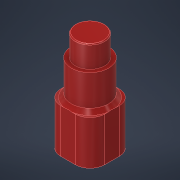
# Autodesk Inventor part: CH_01_0020_servo_shaft_1
Saved by Autodesk Inventor 2022 (Build 260153000, 153)
## iProperties
Created: 2022-03-04
Part Number: CH_01_0020_servo_shaft_1
Material: Ogólny
Document SubType Name: Modeling
Designer: zsamot8
Density: 1 g/cm^3
Appearance: Czerwona
Author: zsamot8
Autodesk Inventor part; units mm, degrees
ref_plane "YZ Plane" through (0, 0, 0) normal (1, 0, 0) x (0, 1, 0)
ref_plane "XZ Plane" through (0, 0, 0) normal (0, 1, 0) x (-1, 0, 0)
ref_plane "XY Plane" through (0, 0, 0) normal (0, 0, 1) x (1, 0, 0)
sketch "Szkic1" plane through (0, 0, 0) normal (0, 1, 0) x (-1, 0, 0)
  line L0 (-2.75, 2.75) -> (2.75, 2.75)
  line L1 (2.75, 2.75) -> (2.75, -2.75)
  line L2 (2.75, -2.75) -> (-2.75, -2.75)
  line L3 (-2.75, -2.75) -> (-2.75, 2.75)
  line L4 (-2.75, 2.75) -> (2.75, -2.75) construction
  line L5 (2.75, 2.75) -> (-2.75, -2.75) construction
  line L6 (-2, 6) -> (2, 6)
  line L7 (6, 2) -> (6, -2)
  line L8 (2, -6) -> (-2, -6)
  line L9 (-6, -2) -> (-6, 2)
  line L10 (-6, 6) -> (6, -6) construction
  line L11 (6, 6) -> (-6, -6) construction
  arc A0 (6, 2) -> (2, 6) centre (2, 2) ccw
  arc A1 (2, -6) -> (6, -2) centre (2, -2) ccw
  arc A2 (-6, -2) -> (-2, -6) centre (-2, -2) ccw
  arc A3 (-2, 6) -> (-6, 2) centre (-2, 2) ccw
  point P0 (0, 0)
  dimension "d0" = 5.5
  dimension "d1" = 12
  dimension "d2" = 4
  constraints: 24 end point, 9 point on line, 8 point on circle, 8 tangent, 4 centre point, 4 midpoint, 4 parallel, 3 equal radius, 3 perpendicular, 2 horizontal
  measures "d0" distance between parallel lines of L2 L0
  measures "d1" distance of L11.start L10.end
  measures "d2" radius of A0
extrude "Wyciągnięcie proste1" add sketch "Szkic1" along normal blind 10
sketch "Szkic2" plane through (0, 10, 0) normal (0, 1, 0) x (1, 0, 0)
  arc A0 (-6, -2) -> (-2, -6) centre (-2, -2) ccw projected
  line L0 (-6, 2) -> (-6, -2) projected
  arc A1 (-2, 6) -> (-6, 2) centre (-2, 2) ccw projected
  line L1 (2, 6) -> (-2, 6) projected
  arc A2 (6, 2) -> (2, 6) centre (2, 2) ccw projected
  line L2 (6, -2) -> (6, 2) projected
  arc A3 (2, -6) -> (6, -2) centre (2, -2) ccw projected
  line L3 (-2, -6) -> (2, -6) projected
extrude "Wyciągnięcie proste2" add sketch "Szkic2" along normal blind 2
sketch "Szkic3" plane through (0, 12, 0) normal (0, 1, 0) x (1, 0, 0)
  circle A0 centre (0, 0) radius 4
  dimension "d7" = 8
  constraints: 1 centre point, 1 coincident
  measures "d7" diameter of A0
extrude "Wyciągnięcie proste3" add sketch "Szkic3" along normal blind 15.45
sketch "Szkic5" plane through (0, 12, 0) normal (0, 1, 0) x (1, 0, 0)
  circle A0 centre (0, 0) radius 5.1
  dimension "d19" = 10.2
  constraints: 1 centre point, 1 coincident
  measures "d19" diameter of A0
extrude "Wyciągnięcie proste4" add sketch "Szkic5" along normal blind 6.15
fillet "Zaokrąglenie2" radius 0.25 1 edges at (-4, 27.45, 0)
chamfer "Faza1" distance 1 angle 45 4 edges at (-2.75, 10, 0) (0, 10, 2.75) (2.75, 10, 0) (0, 10, -2.75)
sketch "Sketch6" plane through (0, 18.15, 0) normal (0, 1, 0) x (1, 0, 0)
  circle A0 centre (0, 0) radius 5.1 projected
  circle A1 centre (0, 0) radius 4 projected
extrude "Extrusion5" add sketch "Sketch6" along normal blind 3.3 contours A0 | A1
chamfer "Chamfer2" distance 1 angle 45 1 edges at (-5.1, 12, 0)
